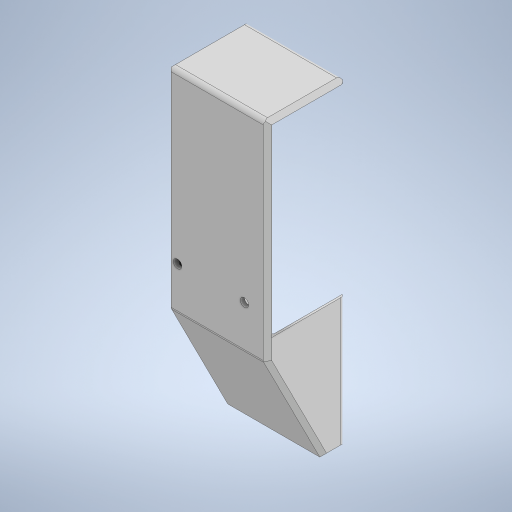
# Autodesk Inventor part: LewyBłotnik
Saved by Autodesk Inventor 2024 (Build 280153000, 153)
## iProperties
Created: 2025-05-22
Part Number: LewyBłotnik
Material: Ogólny
Document SubType Name: Modeling
Designer: Victoria
Density: 1 g/cm^3
Appearance: Domyślna
Author: Victoria
Autodesk Inventor part; units mm, degrees
ref_plane "YZ Plane" through (0, 0, 0) normal (1, 0, 0) x (0, 1, 0)
ref_plane "XZ Plane" through (0, 0, 0) normal (0, 1, 0) x (-1, 0, 0)
ref_plane "XY Plane" through (0, 0, 0) normal (0, 0, 1) x (1, 0, 0)
sketch "Szkic1" plane through (0, 0, 0) normal (0, 0, 1) x (1, 0, 0)
  circle A0 centre (16, 0) radius 2
  circle A1 centre (-16, 0) radius 2
  line L0 (28, -73) -> (-21, -73)
  line L1 (-21, -73) -> (-21, 0)
  line L2 (28, 80) -> (-21, 80)
  line L3 (-21, 80) -> (-21, 0)
  line L4 (28, -73) -> (27, -73)
  line L5 (27, -73) -> (27, 80)
  point P0 (0, 0)
  point P1 (-21, 83.4616)
  dimension "d0" = 4
  dimension "d48" = 1
  constraints: 12 end point, 3 perpendicular, 3 point on line, 2 centre point
  measures "d0" diameter of A0
  measures "d48" distance of L0.start L4.end
extrude "Wyciągnięcie proste1" add sketch "Szkic1" along normal blind 2
sketch "Szkic2" plane through (0, 0, 0) normal (0, 0, -1) x (-1, 0, 0)
  line L0 (21, -73) -> (-27, -73) projected
  line L1 (21, 80) -> (21, -73) projected
  circle A0 centre (16, 0) radius 2 projected
  circle A1 centre (-16, 0) radius 2 projected
  line L2 (19, -10) -> (21, -10)
  line L3 (-27, 80) -> (21, 80) projected
  line L4 (19, -71) -> (-26, -71)
  line L5 (-26, -71) -> (-26, 78)
  line L6 (-26, 78) -> (19, 78)
  line L7 (19, 78) -> (19, -71)
  line L8 (19, 68) -> (21, 68)
  line L9 (-27, -73) -> (-27, 80) projected
  point P0 (0, 0)
  dimension "d10" = 2
  constraints: 12 end point, 3 point on line, 2 perpendicular, 1 other
  measures "d10" distance between parallel lines of L1 L7
extrude "Wyciągnięcie proste2" add sketch "Szkic2" along normal blind 35 contours L0 L9 L3 L1 L8 L7 L6 L5 L4 L2 | L2 L7 L8 L1
sketch "Szkic7" plane through (27, -73, 2) normal (1, 0, 0) x (0, 0, -1)
  line L0 (0, 0) -> (0, 153) projected
  line L1 (37, 0) -> (0, 0) projected
  line L2 (0, 53) -> (27, 0) projected
  point P0 (2, 73)
extrude "Wyciągnięcie proste7" cut sketch "Szkic7" against normal up to surface (48 mm away)
sketch "Szkic9" plane through (27, -73, -35) normal (1, 0, 0) x (0, 0, -1)
  line L0 (-37, 53) -> (-10, 0) projected
  line L1 (0, 0) -> (-10, 0) projected
  line L2 (0, 153) -> (0, 0) projected
  line L3 (0, 153) -> (-37, 153) projected
  line L4 (-37, 53) -> (-37, 153) projected
  line L5 (-10, 0) -> (-8, 0)
  line L6 (0, 0) -> (-10, 0) projected
  line L7 (-37, 53) -> (-35, 53)
  line L8 (-35, 53) -> (-8, 0)
  point P0 (-35, 73)
  point P1 (-8, 0)
  dimension "d54" = 2
  dimension "d55" = 2
  constraints: 6 end point, 1 horizontal, 1 point on line
  measures "d54" distance of L0.end L5.end
  measures "d55" distance of L0.start L7.end
extrude "Wyciągnięcie proste9" add sketch "Szkic9" against normal up to surface (48 mm away) contours L7 L8 L1 L0
chamfer "Faza2" distance 2 angle 45 16 edges at (27, -46.5, -11.5) (27, -73, -30) (27, 30, 2) (27, 80, -16.5) (26, -45.5, -12.9906) (26, -71, -30.4906) (26, 29, 0) (26, 78, -17.5) (-21, -46.5, -11.5) (-21, -73, -30) (-21, 30, 2) (-21, 80, -16.5) (-19, 29, 0) (-19, -45.5, -12.9906) (-19, -71, -30.4906) (-19, 78, -17.5)
fillet "Zaokrąglenie2" radius 2 6 edges at (3, -73, -35) (3, 80, -35) (-21, 3.5, -35) (27, 3.5, -35) (3, -20, 2) (3, 80, 2)
sketch "Szkic10" plane through (-21, -19.5199, 0) normal (-1, 0, 0) x (0, 0, 1)
  line L0 (-33, 97.5199) -> (-33, 88.5199)
  line L1 (-33, 88.5199) -> (-17, 88.5199)
  line L2 (-1, 88.5199) -> (-33, 88.5199)
  line L3 (-17, 88.5199) -> (-17, 1.6565)
  line L4 (-17, 88.5199) -> (-17, 83.5199)
  line L5 (-31, 88.5199) -> (-17, 83.5199)
  line L6 (-17, 83.5199) -> (-3, 88.5199)
  line L7 (-31, 88.5199) -> (-31, 85.5199)
  line L8 (-17, 83.5199) -> (-17, 80.5199)
  line L9 (-17, 80.5199) -> (-31, 85.5199)
  line L10 (-3, 88.5199) -> (-3, 85.5199)
  line L11 (-3, 1.24) -> (-3, 95.5199)
  line L12 (-3, 85.5199) -> (-17, 80.5199)
  line L13 (-17, 77.5199) -> (-3, 82.5199)
  line L14 (-3, 79.5199) -> (-17, 74.5199)
  line L15 (-3, 82.5199) -> (-3, 79.5199)
  line L16 (-31, 82.5199) -> (-17, 77.5199)
  line L17 (-17, 74.5199) -> (-31, 79.5199)
  line L18 (-31, 82.5199) -> (-31, 79.5199)
  line L19 (-17, 71.5199) -> (-3, 76.5199)
  line L20 (-3, 73.5199) -> (-17, 68.5199)
  line L21 (-3, 76.5199) -> (-3, 73.5199)
  line L22 (-31, 76.5199) -> (-17, 71.5199)
  line L23 (-17, 68.5199) -> (-31, 73.5199)
  line L24 (-31, 76.5199) -> (-31, 73.5199)
  line L25 (-17, 65.5199) -> (-3, 70.5199)
  line L26 (-3, 67.5199) -> (-17, 62.5199)
  line L27 (-3, 70.5199) -> (-3, 67.5199)
  line L28 (-31, 70.5199) -> (-17, 65.5199)
  line L29 (-17, 62.5199) -> (-31, 67.5199)
  line L30 (-31, 70.5199) -> (-31, 67.5199)
  line L31 (-17, 59.5199) -> (-3, 64.5199)
  line L32 (-3, 61.5199) -> (-17, 56.5199)
  line L33 (-3, 64.5199) -> (-3, 61.5199)
  line L34 (-31, 64.5199) -> (-17, 59.5199)
  line L35 (-17, 56.5199) -> (-31, 61.5199)
  line L36 (-31, 64.5199) -> (-31, 61.5199)
  line L37 (-17, 53.5199) -> (-3, 58.5199)
  line L38 (-3, 55.5199) -> (-17, 50.5199)
  line L39 (-3, 58.5199) -> (-3, 55.5199)
  line L40 (-31, 58.5199) -> (-17, 53.5199)
  line L41 (-17, 50.5199) -> (-31, 55.5199)
  line L42 (-31, 58.5199) -> (-31, 55.5199)
  line L43 (-17, 47.5199) -> (-3, 52.5199)
  line L44 (-3, 49.5199) -> (-17, 44.5199)
  line L45 (-3, 52.5199) -> (-3, 49.5199)
  line L46 (-31, 52.5199) -> (-17, 47.5199)
  line L47 (-17, 44.5199) -> (-31, 49.5199)
  line L48 (-31, 52.5199) -> (-31, 49.5199)
  line L49 (-17, 41.5199) -> (-3, 46.5199)
  line L50 (-3, 43.5199) -> (-17, 38.5199)
  line L51 (-3, 46.5199) -> (-3, 43.5199)
  line L52 (-31, 46.5199) -> (-17, 41.5199)
  line L53 (-17, 38.5199) -> (-31, 43.5199)
  line L54 (-31, 46.5199) -> (-31, 43.5199)
  line L55 (-17, 35.5199) -> (-3, 40.5199)
  line L56 (-3, 37.5199) -> (-17, 32.5199)
  line L57 (-3, 40.5199) -> (-3, 37.5199)
  line L58 (-31, 40.5199) -> (-17, 35.5199)
  line L59 (-17, 32.5199) -> (-31, 37.5199)
  line L60 (-31, 40.5199) -> (-31, 37.5199)
  line L61 (-17, 29.5199) -> (-3, 34.5199)
  line L62 (-3, 31.5199) -> (-17, 26.5199)
  line L63 (-3, 34.5199) -> (-3, 31.5199)
  line L64 (-31, 34.5199) -> (-17, 29.5199)
  line L65 (-17, 26.5199) -> (-31, 31.5199)
  line L66 (-31, 34.5199) -> (-31, 31.5199)
  line L67 (-33, -51.4801) -> (-33, 97.5199) projected
  line L68 (-26.2257, -51.4801) -> (-33, -51.4801) projected
  line L69 (0, 0) -> (-26.2257, -51.4801) projected
  line L70 (0, 97.5199) -> (0, 0) projected
  line L71 (-33, 97.5199) -> (0, 97.5199) projected
  point P0 (0, 19.5199)
  point P1 (0, 20.5199)
  point P2 (-1, 88.5199)
  point P3 (-3, 1.24)
  point P4 (-3, 95.5199)
  point P5 (-19.3663, 2.045)
  point P6 (-3, -7.0919)
  point P7 (-17, 26.5199)
  point P8 (-3, 40.5199)
  point P9 (-17, 62.5199)
  point P10 (-17, 74.5199)
  dimension "d66" = 16
  dimension "d67" = 5
  dimension "d68" = 3
  dimension "d69" = 3
  dimension "d70" = 3
  dimension "d71" = 6
  constraints: 132 end point, 5 point on line, 1 midpoint, 1 perpendicular, 1 vertical, 121 other
  measures "d66" distance of L2.end L4.start
  measures "d67" distance of L4.start L8.start
  measures "d68" distance of L5.start L9.end
  measures "d69" distance of L8.start L8.end
  measures "d70" distance of L6.end L10.end
  measures "d71" distance of L8.start L16.end
extrude "Wyciągnięcie proste10" cut sketch "Szkic10" against normal blind 10 contours L5 L3 L9 L7 | L6 L10 L12 L3 | L13 L11 L14 L3 | L3 L17 L18 L16 | L19 L11 L20 L3 | L3 L23 L24 L22 | L25 L11 L26 L3 | L3 L29 L30 L28 | L31 L11 L32 L3 | L3 L35 L36 L34 | L37 L11 L38 L3 | L3 L41 L42 L40 | L43 L11 L44 L3 | L3 L47 L48 L46 | L49 L11 L50 L3 | L3 L53 L54 L52 | L55 L11 L56 L3 | L3 L59 L60 L58 | L61 L11 L62 L3 | L3 L65 L66 L64
sketch "Szkic12" plane through (27, -19.5199, 0) normal (1, 0, 0) x (0, 0, -1)
  line L0 (0, 9.52) -> (35, 9.52)
  line L1 (35, 9.52) -> (35, 97.5199)
  line L2 (35, 97.5199) -> (0, 97.5199)
  line L3 (0, 97.5199) -> (0, 9.52)
  point P0 (0, 19.5199)
  constraints: 8 end point, 2 parallel, 1 horizontal, 1 perpendicular
extrude "Wyciągnięcie proste12" cut sketch "Szkic12" against normal blind 10
